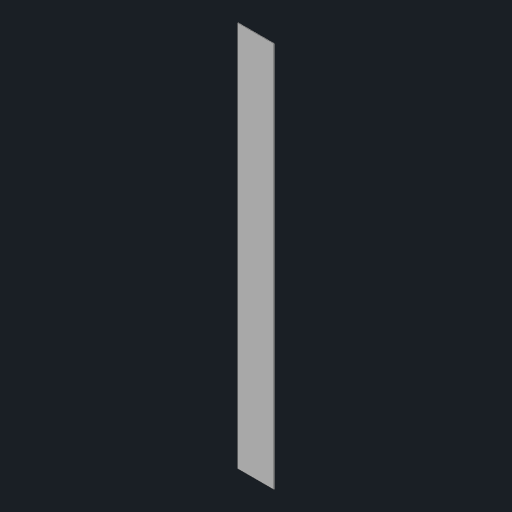
# Autodesk Inventor part: CARCASA_ALUM_8
Saved by Autodesk Inventor 2024.3 (Build 283343000, 343)
## iProperties
Created: 2024-05-15
Part Number: CARCASA_ALUM_8
Material: Generic
Document SubType Name: Sheet Metal
Designer: Niler
Density: 1 g/cm^3
Sheet Metal Rule: Default_mm
Appearance: Default
Author: Niler
Autodesk Inventor part; units mm, degrees
ref_plane "YZ Plane" through (0, 0, 0) normal (1, 0, 0) x (0, 1, 0)
ref_plane "XZ Plane" through (0, 0, 0) normal (0, 1, 0) x (-1, 0, 0)
ref_plane "Work Plane1" through (0, 0, 0) normal (0, 0, 1) x (1, 0, 0)
sketch "Sketch1" plane through (0, 0, 0) normal (0, 0, 1) x (1, 0, 0)
  line L0 (0, -790) -> (0, 230)
  line L1 (0, -810) -> (0, -790)
  line L2 (0, -810) -> (100, -810)
  line L3 (100, -810) -> (100, -560)
  line L4 (10, -560) -> (100, -560)
  line L5 (10, -560) -> (10, 0)
  line L6 (10, 0) -> (100, 0)
  line L7 (100, 0) -> (100, 250)
  line L8 (0, 250) -> (100, 250)
  line L9 (0, 230) -> (0, 250)
  line L10 (100, 0) -> (100, -560)
  point P0 (0, 0)
extrude "Plate1" add sketch "Sketch1" against normal blind 1.5
equation "\"d0\" = Thickness"
equation "\"BendRadius\" = Thickness"
equation "\"BendReliefWidth\" = Thickness"
equation "\"BendReliefDepth\" = 0.5 * Thickness"
equation "\"CornerReliefSize\" = 4 * Thickness"
equation "\"MinimumRemnant\" = 2 * Thickness"
equation "\"TransitionRadius\" = BendRadius"
equation "\"JacobiRadiusSize\" = BendRadius"
equation "\"GapSize\" = Thickness"
equation "\"Thickness\" = 1.5"
body "Solid1"
